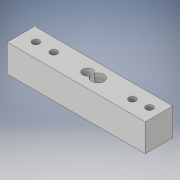
# Autodesk Inventor part: measuring the torque
Saved by Autodesk Inventor 2019 (Build 230136000, 136)
## iProperties
Created: 2020-03-01
Part Number: measuring the torque
Material: Generic
Document SubType Name: Modeling
Designer: VIGNESH
Density: 1 g/cm^3
Appearance: Default
Author: VIGNESH
Autodesk Inventor part; units mm, degrees
ref_plane "YZ Plane" through (0, 0, 0) normal (1, 0, 0) x (0, 1, 0)
ref_plane "XZ Plane" through (0, 0, 0) normal (0, 1, 0) x (-1, 0, 0)
ref_plane "XY Plane" through (0, 0, 0) normal (0, 0, 1) x (1, 0, 0)
sketch "Sketch1" plane through (0, 0, 0) normal (0, 0, 1) x (1, 0, 0)
  line L0 (0, 0) -> (100, 0)
  line L1 (100, 0) -> (100, 20)
  line L2 (100, 20) -> (0, 20)
  line L3 (0, 20) -> (0, 0)
  dimension "d0" = 100
  dimension "d1" = 20
  constraints: 8 end point, 2 parallel, 1 horizontal, 1 perpendicular
  measures "d0" distance of L2.end L1.end
  measures "d1" distance of L1.end L0.end
extrude "Extrusion1" add sketch "Sketch1" along normal blind 20
sketch "Sketch2" plane through (0, 20, 0) normal (0, 1, 0) x (1, 0, 0)
  circle A0 centre (10.3006, -9.5044) radius 3.7411
  circle A1 centre (23.2386, -9.5044) radius 3.8763
  circle A2 centre (92.585, -9.5044) radius 4.8406
  circle A3 centre (81.1397, -10.4639) radius 4.4927
  point P0 (0, 0)
  constraints: 4 centre point
hole "Hole1" at (10.3006, 20, 9.5044) at (23.2386, 20, 9.5044) at (81.1397, 20, 10.4639) at (92.585, 20, 9.5044) direction (0, -1, 0) diameter 5 end through all
sketch "Sketch3" plane through (0, 20, 0) normal (0, 1, 0) x (1, 0, 0)
  point P0 (0, 0)
sketch "Sketch4" plane through (0, 20, 0) normal (0, 1, 0) x (1, 0, 0)
  arc A0 (51.1615, -7.9359) -> (51.1615, -11.2858) centre (47.9614, -9.6108) ccw
  arc A1 (51.1615, -11.2858) -> (51.1615, -7.9359) centre (55.2972, -9.6108) ccw
  point P0 (0, 0)
  constraints: 4 point on circle, 2 centre point
extrude "Extrusion2" cut sketch "Sketch4" along normal mid plane 100
body "Solid1"
